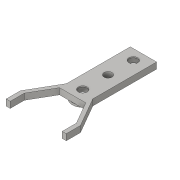
# Autodesk Inventor part: 28_Z_Stage
Saved by Autodesk Inventor 2016 (Build 200138000, 138)
## iProperties
Created: 2017-01-03
Part Number: 28_Z_Stage
Material: Generisch
Document SubType Name: Modeling
Designer: Bene
Density: 1 g/cm^3
Appearance: Vorgabe
Author: Bene
Autodesk Inventor part; units mm, degrees
ref_plane "YZ Plane" through (0, 0, 0) normal (1, 0, 0) x (0, 1, 0)
ref_plane "XZ Plane" through (0, 0, 0) normal (0, 1, 0) x (-1, 0, 0)
ref_plane "XY Plane" through (0, 0, 0) normal (0, 0, 1) x (1, 0, 0)
sketch "Skizze4" plane through (0, 0, 0) normal (0, 0, 1) x (1, 0, 0)
  circle A0 centre (0, 25) radius 4 construction
  circle A1 centre (0, -25) radius 4 construction
  circle A2 centre (0, 0) radius 3 construction
  line L0 (-11.0333, -36.517) -> (-22.869, -57.017) construction
  line L1 (12.638, -36.517) -> (-11.0333, -36.517) construction
  line L2 (24.4737, -57.017) -> (12.638, -36.517) construction
  line L3 (12.638, -77.517) -> (24.4737, -57.017) construction
  circle A3 centre (0.8023, -57.017) radius 18 construction
  line L4 (12.638, -36.517) -> (-11.0333, -36.517) construction
  line L5 (-11.0333, -36.517) -> (-22.869, -57.017) construction
  line L6 (-22.869, -57.017) -> (-11.0334, -77.517) construction
  line L7 (-11.0334, -77.517) -> (12.638, -77.517) construction
  line L8 (12.638, -77.517) -> (24.4737, -57.017) construction
  line L9 (24.4737, -57.017) -> (12.638, -36.517) construction
  circle A4 centre (0, 25) radius 4.3
  circle A5 centre (0, -25) radius 4.3
  circle A6 centre (0, 0) radius 4
  circle A7 centre (0, 25) radius 8 construction
  circle A8 centre (0, -25) radius 8 projected
  circle A9 centre (0, -25) radius 8.3
  circle A10 centre (0, 25) radius 8.3
  line L10 (-13, 35) -> (13, 35)
  line L11 (13, 35) -> (13, -35)
  line L12 (13, -35) -> (-13, -35)
  line L13 (-13, -35) -> (-13, 35)
  line L14 (-13, 35) -> (13, -35) construction
  line L15 (13, 35) -> (-13, -35) construction
  line L16 (-13, -35) -> (-25.7115, -57.017)
  line L17 (-13, -35) -> (12.423, -35) construction
  line L18 (-25.7115, -57.017) -> (-25.7115, -71.017)
  line L19 (-25.7115, -71.017) -> (-29.7115, -71.017)
  line L20 (-29.7115, -71.017) -> (-29.7115, -57.017)
  line L21 (-29.7115, -57.017) -> (-13, -28.0718)
  line L22 (13, -35) -> (25.7115, -57.017)
  line L23 (13, -35) -> (38.423, -35) construction
  line L24 (25.7115, -57.017) -> (25.7115, -71.017)
  line L25 (25.7115, -71.017) -> (29.7115, -71.017)
  line L26 (29.7115, -71.017) -> (29.7115, -57.017)
  line L27 (29.7115, -57.017) -> (13, -28.0718)
  point P0 (0, 0)
  dimension "d22" = 0.3
  dimension "d23" = 0.3
  dimension "d24" = 1
  dimension "d25" = 0.3
  dimension "d26" = 0.3
  dimension "d27" = 26
  dimension "d28" = 70
  dimension "d29" = 120
  dimension "d30" = 14
  dimension "d31" = 4
  dimension "d32" = 90
  dimension "d33" = 60
  dimension "d34" = 4
  dimension "d35" = 90
  dimension "d36" = 150
  dimension "d46" = 12.7115
  dimension "d47" = 0
  constraints: 36 end point, 5 centre point, 5 perpendicular, 3 equal length, 3 horizontal, 2 midpoint, 2 parallel, 2 point on line, 2 vertical
  measures "d22" radial gap between concentric circles of A0 A4
  measures "d23" radial gap between concentric circles of A1 A5
  measures "d24" radial gap between concentric circles of A2 A6
  measures "d25" radial gap between concentric circles of A8 A9
  measures "d26" radial gap between concentric circles of A7 A10
  measures "d27" distance of L11.end L12.end
  measures "d28" distance of L10.end L11.end
  measures "d29" angle of L16 L17
  measures "d30" distance of L16.end L18.end
  measures "d31" distance of L18.end L19.end
  measures "d32" angle of L18 L19
  measures "d33" angle of L22 L23
  measures "d34" distance of L24.end L25.end
  measures "d35" angle of L25 L24
  measures "d36" angle of L27 L26
  measures "d46" distance between parallel lines of L18 L13
  measures "d47" distance between parallel lines of L19 L25
extrude "Extrusion4" add sketch "Skizze4" along normal up to surface (5.1 mm away) contours L10 L11 L12 L13 | L13 L16 L18 L19 L20 L21 | L27 L26 L25 L24 L22 L11
sketch "Skizze5" plane through (-13, -35, 5.1) normal (0, 0, 1) x (1, 0, 0)
  circle A0 centre (13, 60) radius 4 construction
  circle A1 centre (13, 10) radius 4 construction
  circle A2 centre (13, 60) radius 8.3 projected
  circle A3 centre (13, 10) radius 8.3 projected
  circle A4 centre (13, 35) radius 4 projected
  line L0 (26, 0) -> (0, 0) projected
  line L1 (38.7115, -22.017) -> (26, 0) projected
  line L2 (38.7115, -36.017) -> (38.7115, -22.017) projected
  line L3 (42.7115, -36.017) -> (38.7115, -36.017) projected
  line L4 (42.7115, -22.017) -> (42.7115, -36.017) projected
  line L5 (26, 6.9282) -> (42.7115, -22.017) projected
  line L6 (26, 70) -> (26, 6.9282) projected
  line L7 (0, 70) -> (26, 70) projected
  line L8 (0, 6.9282) -> (0, 70) projected
  line L9 (-16.7115, -22.017) -> (0, 6.9282) projected
  line L10 (-16.7115, -36.017) -> (-16.7115, -22.017) projected
  line L11 (-12.7115, -36.017) -> (-16.7115, -36.017) projected
  line L12 (-12.7115, -22.017) -> (-12.7115, -36.017) projected
  line L13 (0, 0) -> (-12.7115, -22.017) projected
  circle A5 centre (13, 60) radius 4.4
  circle A6 centre (13, 10) radius 4.4
  point P0 (13, 35)
  dimension "d39" = 0.4
  dimension "d40" = 0.4
  constraints: 2 centre point
  measures "d39" radial gap between concentric circles of A0 A5
  measures "d40" radial gap between concentric circles of A1 A6
extrude "Extrusion5" add sketch "Skizze5" along normal blind 1 contours A2 | A3 | L0 L13 L12 L11 L10 L9 L8 L7 L6 L5 L4 L3 L2 L1
shell "Wandung1" thickness 2 removed faces 1 at (-11.3529, 9.9806, 0)
sketch "Skizze6" plane through (0, 0, 0) normal (0, 0, -1) x (-1, 0, 0)
  circle A0 centre (0, -25) radius 4.4 projected
  circle A1 centre (0, -25) radius 8.3 projected
  arc A2 (-6.4877, 33) -> (6.4877, 33) centre (0, 25) ccw projected
  circle A3 centre (0, 25) radius 4.4 projected
  circle A4 centre (0, 25) radius 8.3 projected
  arc A5 (6.4877, -33) -> (-6.4877, -33) centre (0, -25) ccw projected
  circle A6 centre (0, -25) radius 10.3
  circle A7 centre (0, 25) radius 10.3
  point P0 (0, 0)
  dimension "d27" = 26
  constraints: 2 coincident, 6 other
extrude "Extrusion6" add sketch "Skizze6" along normal blind 2 contours A7 A2 | A6 A5
